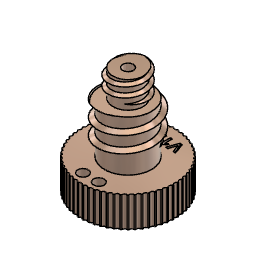
VialThermocoupleFastener_V1.2.0 (Autodesk Fusion 360 design; units mm, degrees)
Autodesk Fusion 360 part; units mm, degrees
note: some values were not read from the file. Chosen so that the rebuilt part matches the saved one: which bodies a step acts on. Set by a fixed rule: which sketch regions a step uses.
sketch "Sketch1" plane through (0, 0, 0) normal (0, 1, 0) x (1, 0, 0)
  circle A0 centre (0, 0) radius 9
  arc A1 (0.148, -8.9988) -> (-0.148, -8.9988) centre (0, -9.0603) ccw
  arc A2 (-0.0491, 8.9999) -> (0.0497, 8.9999) centre (0.0003, 9.0258) ccw
  arc A3 (0.148, -8.9988) -> (-0.148, -8.9988) centre (0, -9.0252) ccw
  arc A4 (0.3504, -8.9932) -> (-0.3525, -8.9931) centre (-0.0011, -9.1863) ccw
  dimension "d1" = 18
  constraint coincident A0.centre origin
  constraint coincident A0 A1.start
  constraint coincident A0 A1.end
  constraint coincident A0 A2.end
  constraint coincident A0 A2.start
  constraint coincident A0 A4.start
  constraint coincident A0 A4.end
  measures "d1" diameter of A0
extrude "Extrude1" add sketch "Sketch1" along normal mid plane 5.7 makes body 1
sketch "Sketch2" plane through (0, 2.85, 0) normal (0, 1, 0) x (-1, 0, 0)
  circle A0 centre (0, 0) radius 9
  circle A1 centre (0, 0) radius 4.425
  circle A2 centre (0, 0) radius 2.85
  dimension "d4" = 8.85
  dimension "d5" = 5.7
  constraint coincident A0.centre A1.centre
  measures "d4" diameter of A1
  measures "d5" diameter of A2
extrude "Extrude2" add sketch "Sketch2" along normal blind 14.5 contours A2 bodies 1
extrude "Extrude3" add sketch "Sketch2" along normal blind 9.5 contours A1 bodies 1
sketch "Sketch3" plane through (0, -2.85, 0) normal (0, -1, 0) x (1, 0, 0)
  circle A0 centre (0, 0) radius 1
  circle A1 centre (1.5, 7) radius 1
  circle A2 centre (-1.5, 7) radius 1
  circle A3 centre (0, 0) radius 9
  dimension "d10" = 2
  dimension "d11" = 2
  dimension "d12" = 2
  measures "d10" diameter of A0
  measures "d11" diameter of A1
  measures "d12" diameter of A2
extrude "Extrude4" cut sketch "Sketch3" against normal through all contours A0 | A1 | A2 bodies 1
extrude "Extrude5" cut sketch "Sketch1" along normal through all and the other way through all contours A0 A3 A4 | A0 A1 | A1 A3 bodies 1
pattern_circular "C-Pattern1" count 60 over 360 about axis through (0, -2.85, 0) along (0, -1, 0) of "Extrude5"
coil "CoilPrimitive1" add diameter 8.85 section triangle out size 1.75 on centre turns 3.5 pitch 3 right hand placed x (-1, 0, 0) y (0, 0, 1) z (0, 1, 0) at (0, 2.85, 0) bodies 1
sketch "Sketch5" plane through (0, 2.85, 0) normal (0, 1, 0) x (-1, 0, 0)
  line L0 (5.3, 0) -> (4.425, 0)
  arc A0 (2.1708, 3.8559) -> (4.425, 0) centre (0, 0) ccw
  circle A1 centre (1.5, 7) radius 1
  circle A2 centre (-1.5, 7) radius 1
  circle A3 centre (0, 0) radius 5.3951
  circle A4 centre (0, 0) radius 4.425
  circle A5 centre (0, 0) radius 2.75
  spline S0 degree 3 poles (2.1708, 3.8559) (2.2571, 3.8266) (2.3426, 3.7945) (2.975, 3.5341) (3.4721, 3.2005) (4.2617, 2.4207) (4.5672, 2) (5.0497, 1.0568) (5.2163, 0.5365) (5.3, 0) knots 0.431144 0.431144 0.431144 0.431144 0.458428 0.458428 0.635267 0.635267 0.789156 0.789156 0.950742 0.950742 0.950742 0.950742
  arc A6 (-1.2885, 8.9073) -> (-0.5894, 8.9807) centre (-0.9591, 9.1361) ccw
  arc A7 (-2.2125, 8.7238) -> (-1.5249, 8.8699) centre (-1.9089, 8.9858) ccw
  arc A8 (-3.1123, 8.4447) -> (-2.4437, 8.6619) centre (-2.8377, 8.737) ccw
  arc A9 (-3.9779, 8.0732) -> (-3.3358, 8.359) centre (-3.7354, 8.3926) ccw
  arc A10 (-4.8, 7.6131) -> (-4.1912, 7.9645) centre (-4.5922, 7.9561) ccw
  arc A11 (-5.5695, 7.0697) -> (-5.0008, 7.4828) centre (-5.3987, 7.4325) ccw
  arc A12 (-6.278, 6.4488) -> (-5.7556, 6.9191) centre (-6.146, 6.8275) ccw
  arc A13 (-6.9177, 5.7572) -> (-6.4473, 6.2795) centre (-6.826, 6.1477) ccw
  arc A14 (-7.4816, 5.0026) -> (-7.0683, 5.5712) centre (-7.4312, 5.4005) ccw
  arc A15 (-7.9635, 4.1932) -> (-7.612, 4.8019) centre (-7.955, 4.5941) ccw
  arc A16 (-8.3582, 3.3378) -> (-8.0722, 3.9799) centre (-8.3917, 3.7374) ccw
  arc A17 (-8.6613, 2.4458) -> (-8.444, 3.1143) centre (-8.7364, 2.8398) ccw
  arc A18 (-8.8695, 1.5271) -> (-8.7233, 2.2146) centre (-8.9853, 1.911) ccw
  arc A19 (-8.9805, 0.5916) -> (-8.907, 1.2906) centre (-9.1359, 0.9613) ccw
  arc A20 (-8.9932, -0.3504) -> (-8.9931, 0.3525) centre (-9.1863, 0.0011) ccw
  arc A21 (-8.9073, -1.2885) -> (-8.9807, -0.5894) centre (-9.1361, -0.9591) ccw
  arc A22 (-8.7238, -2.2125) -> (-8.8699, -1.5249) centre (-8.9858, -1.9089) ccw
  arc A23 (-8.4447, -3.1123) -> (-8.6619, -2.4437) centre (-8.737, -2.8377) ccw
  arc A24 (-8.0732, -3.9779) -> (-8.359, -3.3358) centre (-8.3926, -3.7354) ccw
  arc A25 (-7.6131, -4.8) -> (-7.9645, -4.1912) centre (-7.9561, -4.5922) ccw
  arc A26 (-7.0697, -5.5695) -> (-7.4828, -5.0008) centre (-7.4325, -5.3987) ccw
  arc A27 (-6.4488, -6.278) -> (-6.9191, -5.7556) centre (-6.8275, -6.146) ccw
  arc A28 (-5.7572, -6.9177) -> (-6.2795, -6.4473) centre (-6.1477, -6.826) ccw
  arc A29 (-5.0026, -7.4816) -> (-5.5712, -7.0683) centre (-5.4005, -7.4312) ccw
  arc A30 (-4.1932, -7.9635) -> (-4.8019, -7.612) centre (-4.5941, -7.955) ccw
  arc A31 (-3.3378, -8.3582) -> (-3.9799, -8.0722) centre (-3.7374, -8.3917) ccw
  arc A32 (-2.4458, -8.6613) -> (-3.1143, -8.444) centre (-2.8398, -8.7364) ccw
  arc A33 (-1.5271, -8.8695) -> (-2.2146, -8.7233) centre (-1.911, -8.9853) ccw
  arc A34 (-0.5916, -8.9805) -> (-1.2906, -8.907) centre (-0.9613, -9.1359) ccw
  arc A35 (0.3504, -8.9932) -> (-0.3525, -8.9931) centre (-0.0011, -9.1863) ccw
  arc A36 (1.2885, -8.9073) -> (0.5894, -8.9807) centre (0.9591, -9.1361) ccw
  arc A37 (2.2125, -8.7238) -> (1.5249, -8.8699) centre (1.9089, -8.9858) ccw
  arc A38 (3.1123, -8.4447) -> (2.4437, -8.6619) centre (2.8377, -8.737) ccw
  arc A39 (3.9779, -8.0732) -> (3.3358, -8.359) centre (3.7354, -8.3926) ccw
  arc A40 (4.8, -7.6131) -> (4.1912, -7.9645) centre (4.5922, -7.9561) ccw
  arc A41 (5.5695, -7.0697) -> (5.0008, -7.4828) centre (5.3987, -7.4325) ccw
  arc A42 (6.278, -6.4488) -> (5.7556, -6.9191) centre (6.146, -6.8275) ccw
  arc A43 (6.9177, -5.7572) -> (6.4473, -6.2795) centre (6.826, -6.1477) ccw
  arc A44 (7.4816, -5.0026) -> (7.0683, -5.5712) centre (7.4312, -5.4005) ccw
  arc A45 (7.9635, -4.1932) -> (7.612, -4.8019) centre (7.955, -4.5941) ccw
  arc A46 (8.3582, -3.3378) -> (8.0722, -3.9799) centre (8.3917, -3.7374) ccw
  arc A47 (8.6613, -2.4458) -> (8.444, -3.1143) centre (8.7364, -2.8398) ccw
  arc A48 (8.8695, -1.5271) -> (8.7233, -2.2146) centre (8.9853, -1.911) ccw
  arc A49 (8.9805, -0.5916) -> (8.907, -1.2906) centre (9.1359, -0.9613) ccw
  arc A50 (8.9932, 0.3504) -> (8.9931, -0.3525) centre (9.1863, -0.0011) ccw
  arc A51 (8.9073, 1.2885) -> (8.9807, 0.5894) centre (9.1361, 0.9591) ccw
  arc A52 (8.7238, 2.2125) -> (8.8699, 1.5249) centre (8.9858, 1.9089) ccw
  arc A53 (8.4447, 3.1123) -> (8.6619, 2.4437) centre (8.737, 2.8377) ccw
  arc A54 (8.0732, 3.9779) -> (8.359, 3.3358) centre (8.3926, 3.7354) ccw
  arc A55 (7.6131, 4.8) -> (7.9645, 4.1912) centre (7.9561, 4.5922) ccw
  arc A56 (7.0697, 5.5695) -> (7.4828, 5.0008) centre (7.4325, 5.3987) ccw
  arc A57 (6.4488, 6.278) -> (6.9191, 5.7556) centre (6.8275, 6.146) ccw
  arc A58 (5.7572, 6.9177) -> (6.2795, 6.4473) centre (6.1477, 6.826) ccw
  arc A59 (5.0026, 7.4816) -> (5.5712, 7.0683) centre (5.4005, 7.4312) ccw
  arc A60 (4.1932, 7.9635) -> (4.8019, 7.612) centre (4.5941, 7.955) ccw
  arc A61 (3.3378, 8.3582) -> (3.9799, 8.0722) centre (3.7374, 8.3917) ccw
  arc A62 (2.4458, 8.6613) -> (3.1143, 8.444) centre (2.8398, 8.7364) ccw
  arc A63 (1.5271, 8.8695) -> (2.2146, 8.7233) centre (1.911, 8.9853) ccw
  arc A64 (0.5916, 8.9805) -> (1.2906, 8.907) centre (0.9613, 9.1359) ccw
  arc A65 (-0.3504, 8.9932) -> (0.3525, 8.9931) centre (0.0011, 9.1863) ccw
  arc A66 (-1.2885, 8.9073) -> (-1.5249, 8.8699) centre (0, 0) ccw
  arc A67 (-2.2125, 8.7238) -> (-2.4437, 8.6619) centre (0, 0) ccw
  arc A68 (-3.1123, 8.4447) -> (-3.3358, 8.359) centre (0, 0) ccw
  arc A69 (-3.9779, 8.0732) -> (-4.1912, 7.9645) centre (0, 0) ccw
  arc A70 (-4.8, 7.6131) -> (-5.0008, 7.4828) centre (0, 0) ccw
  arc A71 (-5.5695, 7.0697) -> (-5.7556, 6.9191) centre (0, 0) ccw
  arc A72 (-6.278, 6.4488) -> (-6.4473, 6.2795) centre (0, 0) ccw
  arc A73 (-6.9177, 5.7572) -> (-7.0683, 5.5712) centre (0, 0) ccw
  arc A74 (-7.4816, 5.0026) -> (-7.612, 4.8019) centre (0, 0) ccw
  arc A75 (-7.9635, 4.1932) -> (-8.0722, 3.9799) centre (0, 0) ccw
  arc A76 (-8.3582, 3.3378) -> (-8.444, 3.1143) centre (0, 0) ccw
  arc A77 (-8.6613, 2.4458) -> (-8.7233, 2.2146) centre (0, 0) ccw
  arc A78 (-8.8695, 1.5271) -> (-8.907, 1.2906) centre (0, 0) ccw
  arc A79 (-8.9805, 0.5916) -> (-8.9931, 0.3525) centre (0, 0) ccw
  arc A80 (-8.9932, -0.3504) -> (-8.9807, -0.5894) centre (0, 0) ccw
  arc A81 (-8.9073, -1.2885) -> (-8.8699, -1.5249) centre (0, 0) ccw
  arc A82 (-8.7238, -2.2125) -> (-8.6619, -2.4437) centre (0, 0) ccw
  arc A83 (-8.4447, -3.1123) -> (-8.359, -3.3358) centre (0, 0) ccw
  arc A84 (-8.0732, -3.9779) -> (-7.9645, -4.1912) centre (0, 0) ccw
  arc A85 (-7.6131, -4.8) -> (-7.4828, -5.0008) centre (0, 0) ccw
  arc A86 (-7.0697, -5.5695) -> (-6.9191, -5.7556) centre (0, 0) ccw
  arc A87 (-6.4488, -6.278) -> (-6.2795, -6.4473) centre (0, 0) ccw
  arc A88 (-5.7572, -6.9177) -> (-5.5712, -7.0683) centre (0, 0) ccw
  arc A89 (-5.0026, -7.4816) -> (-4.8019, -7.612) centre (0, 0) ccw
  arc A90 (-4.1932, -7.9635) -> (-3.9799, -8.0722) centre (0, 0) ccw
  arc A91 (-3.3378, -8.3582) -> (-3.1143, -8.444) centre (0, 0) ccw
  arc A92 (-2.4458, -8.6613) -> (-2.2146, -8.7233) centre (0, 0) ccw
  arc A93 (-1.5271, -8.8695) -> (-1.2906, -8.907) centre (0, 0) ccw
  arc A94 (-0.5916, -8.9805) -> (-0.3525, -8.9931) centre (0, 0) ccw
  arc A95 (0.3504, -8.9932) -> (0.5894, -8.9807) centre (0, 0) ccw
  arc A96 (1.2885, -8.9073) -> (1.5249, -8.8699) centre (0, 0) ccw
  arc A97 (2.2125, -8.7238) -> (2.4437, -8.6619) centre (0, 0) ccw
  arc A98 (3.1123, -8.4447) -> (3.3358, -8.359) centre (0, 0) ccw
  arc A99 (3.9779, -8.0732) -> (4.1912, -7.9645) centre (0, 0) ccw
  arc A100 (4.8, -7.6131) -> (5.0008, -7.4828) centre (0, 0) ccw
  arc A101 (5.5695, -7.0697) -> (5.7556, -6.9191) centre (0, 0) ccw
  arc A102 (6.278, -6.4488) -> (6.4473, -6.2795) centre (0, 0) ccw
  arc A103 (6.9177, -5.7572) -> (7.0683, -5.5712) centre (0, 0) ccw
  arc A104 (7.4816, -5.0026) -> (7.612, -4.8019) centre (0, 0) ccw
  arc A105 (7.9635, -4.1932) -> (8.0722, -3.9799) centre (0, 0) ccw
  arc A106 (8.3582, -3.3378) -> (8.444, -3.1143) centre (0, 0) ccw
  arc A107 (8.6613, -2.4458) -> (8.7233, -2.2146) centre (0, 0) ccw
  arc A108 (8.8695, -1.5271) -> (8.907, -1.2906) centre (0, 0) ccw
  arc A109 (8.9805, -0.5916) -> (8.9931, -0.3525) centre (0, 0) ccw
  arc A110 (8.9932, 0.3504) -> (8.9807, 0.5894) centre (0, 0) ccw
  arc A111 (8.9073, 1.2885) -> (8.8699, 1.5249) centre (0, 0) ccw
  arc A112 (8.7238, 2.2125) -> (8.6619, 2.4437) centre (0, 0) ccw
  arc A113 (8.4447, 3.1123) -> (8.359, 3.3358) centre (0, 0) ccw
  arc A114 (8.0732, 3.9779) -> (7.9645, 4.1912) centre (0, 0) ccw
  arc A115 (7.6131, 4.8) -> (7.4828, 5.0008) centre (0, 0) ccw
  arc A116 (7.0697, 5.5695) -> (6.9191, 5.7556) centre (0, 0) ccw
  arc A117 (6.4488, 6.278) -> (6.2795, 6.4473) centre (0, 0) ccw
  arc A118 (5.7572, 6.9177) -> (5.5712, 7.0683) centre (0, 0) ccw
  arc A119 (5.0026, 7.4816) -> (4.8019, 7.612) centre (0, 0) ccw
  arc A120 (4.1932, 7.9635) -> (3.9799, 8.0722) centre (0, 0) ccw
  arc A121 (3.3378, 8.3582) -> (3.1143, 8.444) centre (0, 0) ccw
  arc A122 (2.4458, 8.6613) -> (2.2146, 8.7233) centre (0, 0) ccw
  arc A123 (1.5271, 8.8695) -> (1.2906, 8.907) centre (0, 0) ccw
  arc A124 (0.5916, 8.9805) -> (0.3525, 8.9931) centre (0, 0) ccw
  arc A125 (-0.3504, 8.9932) -> (-0.5894, 8.9807) centre (0, 0) ccw
  dimension "d26" = 8.85
  dimension "d32" = 5.5
  constraint coincident A0.centre A3.centre
  constraint concentric A3 A4
  constraint concentric A4 A5
  measures "d26" diameter of A4
  measures "d32" diameter of A5
extrude "Extrude6" cut sketch "Sketch5" along normal blind 2.25 contours L0 A4 S0 | A3 bodies 1
extrude "Extrude10" cut sketch "Sketch2" along normal blind 2 from surface at 9.5 contours A0 | A1 bodies 1 makes body 2 at (-3.3173, -2.85, 3.9459)
coil "CoilPrimitive4" add diameter 5.7 section triangle out size 1.3 on centre turns 3 pitch 1.8 right hand placed x (-1, 0, 0) y (0, 0, 1) z (0, 1, 0) at (0, 12.35, 0) bodies 2
extrude "Extrude8" cut sketch "Sketch2" along normal blind 1 from surface at 9.5 contours A1 bodies 2
extrude "Extrude11" cut sketch "Sketch2" along normal blind 2 from surface at 14.5 contours A1 | A2 bodies 2
delete_body "RemoveBody1" bodies 1
sketch "Sketch17" plane through (0, 2.85, 0) normal (0, 1, 0) x (-1, 0, 0)
  circle A0 centre (0, 0) radius 4.425
  circle A1 centre (-1.5, 7) radius 1
  circle A2 centre (1.5, 7) radius 1
  arc A3 (-1.2885, 8.9073) -> (-0.5894, 8.9807) centre (-0.9591, 9.1361) ccw
  arc A4 (-1.2885, 8.9073) -> (-1.5249, 8.8699) centre (0, 0) ccw
  arc A5 (-2.2125, 8.7238) -> (-1.5249, 8.8699) centre (-1.9089, 8.9858) ccw
  arc A6 (-2.2125, 8.7238) -> (-2.4437, 8.6619) centre (0, 0) ccw
  arc A7 (-3.1123, 8.4447) -> (-2.4437, 8.6619) centre (-2.8377, 8.737) ccw
  arc A8 (-3.1123, 8.4447) -> (-3.3358, 8.359) centre (0, 0) ccw
  arc A9 (-3.9779, 8.0732) -> (-3.3358, 8.359) centre (-3.7354, 8.3926) ccw
  arc A10 (-3.9779, 8.0732) -> (-4.1912, 7.9645) centre (0, 0) ccw
  arc A11 (-4.8, 7.6131) -> (-4.1912, 7.9645) centre (-4.5922, 7.9561) ccw
  arc A12 (-4.8, 7.6131) -> (-5.0008, 7.4828) centre (0, 0) ccw
  arc A13 (-5.5695, 7.0697) -> (-5.0008, 7.4828) centre (-5.3987, 7.4325) ccw
  arc A14 (-5.5695, 7.0697) -> (-5.7556, 6.9191) centre (0, 0) ccw
  arc A15 (-6.278, 6.4488) -> (-5.7556, 6.9191) centre (-6.146, 6.8275) ccw
  arc A16 (-6.278, 6.4488) -> (-6.4473, 6.2795) centre (0, 0) ccw
  arc A17 (-6.9177, 5.7572) -> (-6.4473, 6.2795) centre (-6.826, 6.1477) ccw
  arc A18 (-6.9177, 5.7572) -> (-7.0683, 5.5712) centre (0, 0) ccw
  arc A19 (-7.4816, 5.0026) -> (-7.0683, 5.5712) centre (-7.4312, 5.4005) ccw
  arc A20 (-7.4816, 5.0026) -> (-7.612, 4.8019) centre (0, 0) ccw
  arc A21 (-7.9635, 4.1932) -> (-7.612, 4.8019) centre (-7.955, 4.5941) ccw
  arc A22 (-7.9635, 4.1932) -> (-8.0722, 3.9799) centre (0, 0) ccw
  arc A23 (-8.3582, 3.3378) -> (-8.0722, 3.9799) centre (-8.3917, 3.7374) ccw
  arc A24 (-8.3582, 3.3378) -> (-8.444, 3.1143) centre (0, 0) ccw
  arc A25 (-8.6613, 2.4458) -> (-8.444, 3.1143) centre (-8.7364, 2.8398) ccw
  arc A26 (-8.6613, 2.4458) -> (-8.7233, 2.2146) centre (0, 0) ccw
  arc A27 (-8.8695, 1.5271) -> (-8.7233, 2.2146) centre (-8.9853, 1.911) ccw
  arc A28 (-8.8695, 1.5271) -> (-8.907, 1.2906) centre (0, 0) ccw
  arc A29 (-8.9805, 0.5916) -> (-8.907, 1.2906) centre (-9.1359, 0.9613) ccw
  arc A30 (-8.9805, 0.5916) -> (-8.9931, 0.3525) centre (0, 0) ccw
  arc A31 (-8.9932, -0.3504) -> (-8.9931, 0.3525) centre (-9.1863, 0.0011) ccw
  arc A32 (-8.9932, -0.3504) -> (-8.9807, -0.5894) centre (0, 0) ccw
  arc A33 (-8.9073, -1.2885) -> (-8.9807, -0.5894) centre (-9.1361, -0.9591) ccw
  arc A34 (-8.9073, -1.2885) -> (-8.8699, -1.5249) centre (0, 0) ccw
  arc A35 (-8.7238, -2.2125) -> (-8.8699, -1.5249) centre (-8.9858, -1.9089) ccw
  arc A36 (-8.7238, -2.2125) -> (-8.6619, -2.4437) centre (0, 0) ccw
  arc A37 (-8.4447, -3.1123) -> (-8.6619, -2.4437) centre (-8.737, -2.8377) ccw
  arc A38 (-8.4447, -3.1123) -> (-8.359, -3.3358) centre (0, 0) ccw
  arc A39 (-8.0732, -3.9779) -> (-8.359, -3.3358) centre (-8.3926, -3.7354) ccw
  arc A40 (-8.0732, -3.9779) -> (-7.9645, -4.1912) centre (0, 0) ccw
  arc A41 (-7.6131, -4.8) -> (-7.9645, -4.1912) centre (-7.9561, -4.5922) ccw
  arc A42 (-7.6131, -4.8) -> (-7.4828, -5.0008) centre (0, 0) ccw
  arc A43 (-7.0697, -5.5695) -> (-7.4828, -5.0008) centre (-7.4325, -5.3987) ccw
  arc A44 (-7.0697, -5.5695) -> (-6.9191, -5.7556) centre (0, 0) ccw
  arc A45 (-6.4488, -6.278) -> (-6.9191, -5.7556) centre (-6.8275, -6.146) ccw
  arc A46 (-6.4488, -6.278) -> (-6.2795, -6.4473) centre (0, 0) ccw
  arc A47 (-5.7572, -6.9177) -> (-6.2795, -6.4473) centre (-6.1477, -6.826) ccw
  arc A48 (-5.7572, -6.9177) -> (-5.5712, -7.0683) centre (0, 0) ccw
  arc A49 (-5.0026, -7.4816) -> (-5.5712, -7.0683) centre (-5.4005, -7.4312) ccw
  arc A50 (-5.0026, -7.4816) -> (-4.8019, -7.612) centre (0, 0) ccw
  arc A51 (-4.1932, -7.9635) -> (-4.8019, -7.612) centre (-4.5941, -7.955) ccw
  arc A52 (-4.1932, -7.9635) -> (-3.9799, -8.0722) centre (0, 0) ccw
  arc A53 (-3.3378, -8.3582) -> (-3.9799, -8.0722) centre (-3.7374, -8.3917) ccw
  arc A54 (-3.3378, -8.3582) -> (-3.1143, -8.444) centre (0, 0) ccw
  arc A55 (-2.4458, -8.6613) -> (-3.1143, -8.444) centre (-2.8398, -8.7364) ccw
  arc A56 (-2.4458, -8.6613) -> (-2.2146, -8.7233) centre (0, 0) ccw
  arc A57 (-1.5271, -8.8695) -> (-2.2146, -8.7233) centre (-1.911, -8.9853) ccw
  arc A58 (-1.5271, -8.8695) -> (-1.2906, -8.907) centre (0, 0) ccw
  arc A59 (-0.5916, -8.9805) -> (-1.2906, -8.907) centre (-0.9613, -9.1359) ccw
  arc A60 (-0.5916, -8.9805) -> (-0.3525, -8.9931) centre (0, 0) ccw
  arc A61 (0.3504, -8.9932) -> (-0.3525, -8.9931) centre (-0.0011, -9.1863) ccw
  arc A62 (0.3504, -8.9932) -> (0.5894, -8.9807) centre (0, 0) ccw
  arc A63 (1.2885, -8.9073) -> (0.5894, -8.9807) centre (0.9591, -9.1361) ccw
  arc A64 (1.2885, -8.9073) -> (1.5249, -8.8699) centre (0, 0) ccw
  arc A65 (2.2125, -8.7238) -> (1.5249, -8.8699) centre (1.9089, -8.9858) ccw
  arc A66 (2.2125, -8.7238) -> (2.4437, -8.6619) centre (0, 0) ccw
  arc A67 (3.1123, -8.4447) -> (2.4437, -8.6619) centre (2.8377, -8.737) ccw
  arc A68 (3.1123, -8.4447) -> (3.3358, -8.359) centre (0, 0) ccw
  arc A69 (3.9779, -8.0732) -> (3.3358, -8.359) centre (3.7354, -8.3926) ccw
  arc A70 (3.9779, -8.0732) -> (4.1912, -7.9645) centre (0, 0) ccw
  arc A71 (4.8, -7.6131) -> (4.1912, -7.9645) centre (4.5922, -7.9561) ccw
  arc A72 (4.8, -7.6131) -> (5.0008, -7.4828) centre (0, 0) ccw
  arc A73 (5.5695, -7.0697) -> (5.0008, -7.4828) centre (5.3987, -7.4325) ccw
  arc A74 (5.5695, -7.0697) -> (5.7556, -6.9191) centre (0, 0) ccw
  arc A75 (6.278, -6.4488) -> (5.7556, -6.9191) centre (6.146, -6.8275) ccw
  arc A76 (6.278, -6.4488) -> (6.4473, -6.2795) centre (0, 0) ccw
  arc A77 (6.9177, -5.7572) -> (6.4473, -6.2795) centre (6.826, -6.1477) ccw
  arc A78 (6.9177, -5.7572) -> (7.0683, -5.5712) centre (0, 0) ccw
  arc A79 (7.4816, -5.0026) -> (7.0683, -5.5712) centre (7.4312, -5.4005) ccw
  arc A80 (7.4816, -5.0026) -> (7.612, -4.8019) centre (0, 0) ccw
  arc A81 (7.9635, -4.1932) -> (7.612, -4.8019) centre (7.955, -4.5941) ccw
  arc A82 (7.9635, -4.1932) -> (8.0722, -3.9799) centre (0, 0) ccw
  arc A83 (8.3582, -3.3378) -> (8.0722, -3.9799) centre (8.3917, -3.7374) ccw
  arc A84 (8.3582, -3.3378) -> (8.444, -3.1143) centre (0, 0) ccw
  arc A85 (8.6613, -2.4458) -> (8.444, -3.1143) centre (8.7364, -2.8398) ccw
  arc A86 (8.6613, -2.4458) -> (8.7233, -2.2146) centre (0, 0) ccw
  arc A87 (8.8695, -1.5271) -> (8.7233, -2.2146) centre (8.9853, -1.911) ccw
  arc A88 (8.8695, -1.5271) -> (8.907, -1.2906) centre (0, 0) ccw
  arc A89 (8.9805, -0.5916) -> (8.907, -1.2906) centre (9.1359, -0.9613) ccw
  arc A90 (8.9805, -0.5916) -> (8.9931, -0.3525) centre (0, 0) ccw
  arc A91 (8.9932, 0.3504) -> (8.9931, -0.3525) centre (9.1863, -0.0011) ccw
  arc A92 (8.9932, 0.3504) -> (8.9807, 0.5894) centre (0, 0) ccw
  arc A93 (8.9073, 1.2885) -> (8.9807, 0.5894) centre (9.1361, 0.9591) ccw
  arc A94 (8.9073, 1.2885) -> (8.8699, 1.5249) centre (0, 0) ccw
  arc A95 (8.7238, 2.2125) -> (8.8699, 1.5249) centre (8.9858, 1.9089) ccw
  arc A96 (8.7238, 2.2125) -> (8.6619, 2.4437) centre (0, 0) ccw
  arc A97 (8.4447, 3.1123) -> (8.6619, 2.4437) centre (8.737, 2.8377) ccw
  arc A98 (8.4447, 3.1123) -> (8.359, 3.3358) centre (0, 0) ccw
  arc A99 (8.0732, 3.9779) -> (8.359, 3.3358) centre (8.3926, 3.7354) ccw
  arc A100 (8.0732, 3.9779) -> (7.9645, 4.1912) centre (0, 0) ccw
  arc A101 (7.6131, 4.8) -> (7.9645, 4.1912) centre (7.9561, 4.5922) ccw
  arc A102 (7.6131, 4.8) -> (7.4828, 5.0008) centre (0, 0) ccw
  arc A103 (7.0697, 5.5695) -> (7.4828, 5.0008) centre (7.4325, 5.3987) ccw
  arc A104 (7.0697, 5.5695) -> (6.9191, 5.7556) centre (0, 0) ccw
  arc A105 (6.4488, 6.278) -> (6.9191, 5.7556) centre (6.8275, 6.146) ccw
  arc A106 (6.4488, 6.278) -> (6.2795, 6.4473) centre (0, 0) ccw
  arc A107 (5.7572, 6.9177) -> (6.2795, 6.4473) centre (6.1477, 6.826) ccw
  arc A108 (5.7572, 6.9177) -> (5.5712, 7.0683) centre (0, 0) ccw
  arc A109 (5.0026, 7.4816) -> (5.5712, 7.0683) centre (5.4005, 7.4312) ccw
  arc A110 (5.0026, 7.4816) -> (4.8019, 7.612) centre (0, 0) ccw
  arc A111 (4.1932, 7.9635) -> (4.8019, 7.612) centre (4.5941, 7.955) ccw
  arc A112 (4.1932, 7.9635) -> (3.9799, 8.0722) centre (0, 0) ccw
  arc A113 (3.3378, 8.3582) -> (3.9799, 8.0722) centre (3.7374, 8.3917) ccw
  arc A114 (3.3378, 8.3582) -> (3.1143, 8.444) centre (0, 0) ccw
  arc A115 (2.4458, 8.6613) -> (3.1143, 8.444) centre (2.8398, 8.7364) ccw
  arc A116 (2.4458, 8.6613) -> (2.2146, 8.7233) centre (0, 0) ccw
  arc A117 (1.5271, 8.8695) -> (2.2146, 8.7233) centre (1.911, 8.9853) ccw
  arc A118 (1.5271, 8.8695) -> (1.2906, 8.907) centre (0, 0) ccw
  arc A119 (0.5916, 8.9805) -> (1.2906, 8.907) centre (0.9613, 9.1359) ccw
  arc A120 (0.5916, 8.9805) -> (0.3525, 8.9931) centre (0, 0) ccw
  arc A121 (-0.3504, 8.9932) -> (0.3525, 8.9931) centre (0.0011, 9.1863) ccw
  arc A122 (-0.3504, 8.9932) -> (-0.5894, 8.9807) centre (0, 0) ccw
  line L0 (-4, -7) -> (4, -7) construction
  line L1 (4, -7) -> (4, -5) construction
  line L2 (4, -5) -> (-4, -5) construction
  line L3 (-4, -5) -> (-4, -7) construction
  dimension "d66" = 2
  text T0 "V1.2.0" font "Arial" height 2 bold align centre top in box 8 x 2 at (-4, -7) x (1, 0) y (0, 1) spacing 1
extrude "Extrude13" cut sketch "Sketch17" against normal blind 0.5 text T0 bodies 2
named bodies: "VTF"
